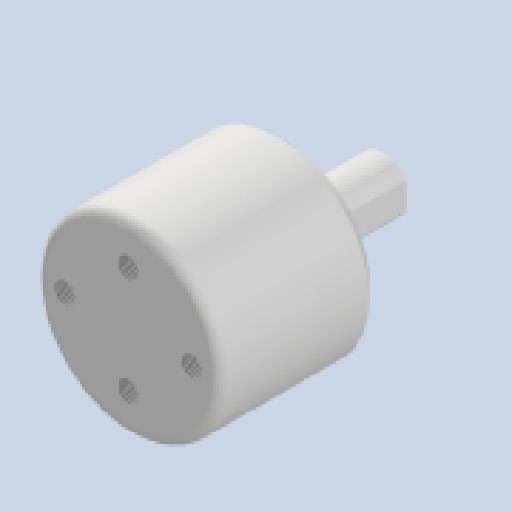
# Autodesk Inventor part: motor
Saved by Autodesk Inventor 2024 (Build 280153000, 153)
## iProperties
Created: 2024-01-11
Part Number: motor
Material: Generic
Document SubType Name: Modeling
Designer: mirun
Density: 1 g/cm^3
Appearance: Default
Author: mirun
Autodesk Inventor part; units mm, degrees
ref_plane "YZ Plane" through (0, 0, 0) normal (1, 0, 0) x (0, 1, 0)
ref_plane "XZ Plane" through (0, 0, 0) normal (0, 1, 0) x (-1, 0, 0)
ref_plane "XY Plane" through (0, 0, 0) normal (0, 0, 1) x (1, 0, 0)
sketch "Sketch1" plane through (0, 0, 0) normal (0, 0, 1) x (1, 0, 0)
  circle A0 centre (0, 0) radius 13.9
  dimension "d0" = 27.8
  constraints: 1 centre point, 1 coincident
  measures "d0" diameter of A0
extrude "Extrusion1" add sketch "Sketch1" along normal blind 24
fillet "Fillet1" radius 1.5 1 edges at (-13.9, 0, 24)
chamfer "Chamfer1" distance 2 angle 45 1 edges at (-13.9, 0, 0)
sketch "Sketch2" plane through (0, 0, 0) normal (0, 0, -1) x (-1, 0, 0)
  circle A0 centre (0, 0) radius 11.9 construction
  circle A1 centre (0, 0) radius 3.94
  line L0 (0, 0) -> (0, -2.6934)
  line L1 (3.4, -1.9909) -> (3.4, 1.9909)
  line L2 (-3.4, -1.9909) -> (-3.4, 1.9909)
  point P0 (0, -1.3467)
  dimension "d7" = 7.88
  dimension "d8" = 6.8
  constraints: 6 end point, 2 point on circle, 2 symmetric about line, 2 vertical, 1 centre point, 1 coincident, 1 midpoint
  measures "d7" diameter of A1
  measures "d8" diameter of L1 point (0, -1.347)
extrude "Extrusion2" add sketch "Sketch2" along normal blind 14 contours L1 A1 L2
sketch "Sketch3" plane through (0, 0, 24) normal (0, 0, 1) x (1, 0, 0)
  circle A0 centre (0, 0) radius 12.4 construction
  line L0 (0, 0) -> (0, 10.8794)
  line L1 (0, 0) -> (9.5, 0)
  circle A1 centre (9.5, 0) radius 1.5
  circle A2 centre (0, 8) radius 1.5
  circle A3 centre (-9.5, 0) radius 1.5
  circle A4 centre (0, -8) radius 1.5
  dimension "d11" = 8
  dimension "d12" = 9.5
  dimension "d13" = 3
  dimension "d14" = 3
  constraints: 5 end point, 4 centre point, 2 coincident, 2 symmetric about line, 1 horizontal, 1 point on line, 1 vertical, 2 other
  measures "d11" distance of L0.start point (0, 8)
  measures "d12" distance of L1.end L0.start
  measures "d13" diameter of A1
  measures "d14" diameter of A2
extrude "Extrusion3" cut sketch "Sketch3" against normal blind 4
thread "Thread1" size "M3x0.5" class "6H" standard "ANSI Metric M Profile" length 30
thread "Thread2" size "M3x0.5" class "6H" standard "ANSI Metric M Profile" length 30
thread "Thread3" size "M3x0.5" class "6H" standard "ANSI Metric M Profile" length 30
thread "Thread4" size "M3x0.5" class "6H" standard "ANSI Metric M Profile" length 30
body "Solid1"
